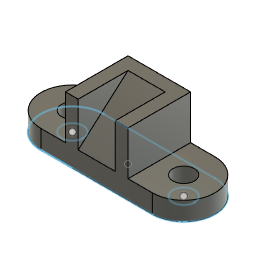
A2 (Autodesk Fusion 360 design; units mm, degrees)
Autodesk Fusion 360 part; units mm, degrees
sketch "Bottom Part" plane through (0, 0, 0) normal (0, 1, 0) x (1, 0, 0)
  line L0 (-57, -32) -> (57, -32)
  line L1 (57, 32) -> (-57, 32)
  circle A0 centre (57, 0) radius 11
  circle A1 centre (-57, 0) radius 11
  arc A2 (-57, 32) -> (-57, -32) centre (-57, 0) ccw
  arc A3 (-57, 32) -> (-57, -32) centre (-57, 0) ccw
  arc A4 (57, -32) -> (57, 32) centre (57, 0) ccw
  dimension "d1" = 114
  dimension "d2" = 64
  dimension "d3" = 32
  dimension "d4" = 32
  dimension "d5" = 22
  dimension "d6" = 22
  constraint horizontal L0
  constraint parallel L0 L1
  constraint concentric A0 A4
  constraint concentric A1 A2
  measures "d1" distance of L1.start L1.end
  measures "d2" distance of L0.end L1.start
  measures "d3" radius of A3
  measures "d4" radius of A2
  measures "d5" diameter of A0
  measures "d6" diameter of A1
extrude "Extrude1" add sketch "Bottom Part" along normal blind 19
sketch "Vertical Part" plane through (0, 19, 0) normal (0, 1, 0) x (-1, 0, 0)
  circle A0 centre (57, 0) radius 11
  circle A1 centre (-57, 0) radius 11
  arc A2 (-57, 32) -> (-57, -32) centre (-57, 0) ccw
  line L0 (-57, -32) -> (57, -32)
  arc A3 (57, -32) -> (57, 32) centre (57, 0) ccw
  line L1 (57, 32) -> (-57, 32)
  line L2 (-32, -32) -> (32, -32)
  line L3 (32, -32) -> (32, 32)
  line L4 (32, 32) -> (-32, 32)
  line L5 (-32, 32) -> (-32, -32)
  line L6 (-32, -32) -> (32, 32) construction
  line L7 (32, -32) -> (-32, 32) construction
  line L8 (19, 32) -> (-19, 32)
  line L9 (-19, 32) -> (-19, -19)
  line L10 (-19, -19) -> (19, -19)
  line L11 (19, -19) -> (19, 32)
  dimension "d9" = 64
  dimension "d10" = 64
  dimension "d11" = 38
  dimension "d12" = 51
  dimension "d13" = 13
  constraint horizontal L2
  constraint perpendicular L2 L3
  constraint parallel L2 L4
  constraint parallel L3 L5
  constraint coincident L6 origin
  constraint coincident L7 origin
  constraint horizontal L8
  constraint vertical L9
  constraint horizontal L10
  constraint vertical L11
  constraint coincident L4 L8.start
  measures "d9" distance of L3.end L4.end
  measures "d10" distance of L2.end L3.end
  measures "d11" distance of L8.start L8.end
  measures "d12" distance of L8.start L10.end
  measures "d13" distance of L3 L11
extrude "Extrude2" add sketch "Vertical Part" along normal blind 45 contours L1 L4 L8 L9 L10 L11
chamfer "Chamfer2" distance 51 distance2 45 1 edges at (0, 64, 32) measured on face at (6.3333, 64, 15)
extrude "Extrude4" add sketch "Vertical Part" along normal blind 45 contours L0 L1 L2 L3 L4 L5 L9 L10 L11
equation "d14 = 64 mm - 19 mm"
named bodies: "A2"
